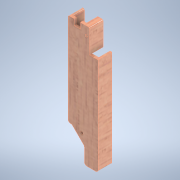
# Autodesk Inventor part: Case
Saved by Autodesk Inventor 2021 (Build 250183000, 183)
## iProperties
Created: 2021-02-15
Part Number: Case
Material: Holz (Eiche)
Document SubType Name: Modeling
Designer: nostrabis
Density: 0.76 g/cm^3
Appearance: Weißeiche - natur - mittlerer Glanz
Mass: 6.60677 g
Surface Area: 82.7336 cm^2
Volume: 8.69312 cm^3
Author: nostrabis
Autodesk Inventor part; units mm, degrees
ref_plane "YZ Plane" through (0, 0, 0) normal (1, 0, 0) x (0, 1, 0)
ref_plane "XZ Plane" through (0, 0, 0) normal (0, 1, 0) x (-1, 0, 0)
sketch "Skizze1" plane through (0, 0, 0) normal (0, 0, 1) x (1, 0, 0)
  point P0 (0, 0)
ref_plane "Arbeitsebene1" through (0, 0, 0) normal (0, 0, 1) x (1, 0, 0)
sketch "Skizze2" plane through (0, 0, 0) normal (0, 0, 1) x (1, 0, 0)
  line L0 (-10, -0.5) -> (-12, -0.5) projected
  line L1 (-12, -0.5) -> (-12, -23.5) projected
  arc A0 (-12, -23.5) -> (-10, -25.5) centre (-10, -23.5) ccw projected
  line L2 (-10, -25.5) -> (-9.8284, -25.5) projected
  arc A1 (-8.4142, -26.0858) -> (-9.8284, -25.5) centre (-9.8284, -27.5) ccw projected
  line L3 (0.4142, -34.9142) -> (-8.4142, -26.0858) projected
  arc A2 (1, -36.3284) -> (0.4142, -34.9142) centre (-1, -36.3284) ccw projected
  line L4 (1, -36.3284) -> (1, -46.5) projected
  arc A3 (1, -46.5) -> (3, -48.5) centre (3, -46.5) ccw projected
  line L5 (3, -48.5) -> (10, -48.5) projected
  arc A4 (10, -48.5) -> (12, -46.5) centre (10, -46.5) ccw projected
  line L6 (12, -46.5) -> (12, 31.5) projected
  line L7 (11, 32.5) -> (10, 32.5) projected
  line L8 (10, 32.5) -> (10, -46.5) projected
  line L9 (10, -46.5) -> (3, -46.5) projected
  line L10 (3, -46.5) -> (3, -23.5) projected
  line L11 (3, -23.5) -> (-10, -23.5) projected
  line L12 (-10, -23.5) -> (-10, -0.5) projected
  arc A5 (1, 48.5) -> (0, 47.5) centre (1, 47.5) ccw projected
  line L13 (0, 47.5) -> (0, 32.5) projected
  line L14 (0, 32.5) -> (5, 32.5) projected
  line L15 (5, 32.5) -> (5, 47.5) projected
  arc A6 (5, 47.5) -> (4, 48.5) centre (4, 47.5) ccw projected
  line L16 (4, 48.5) -> (1, 48.5) projected
  line L17 (-12, 12.5) -> (-10, 12.5) projected
  line L18 (-10, 12.5) -> (-10, 47.5) projected
  arc A7 (-10, 47.5) -> (-12, 47.5) centre (-11, 47.5) ccw projected
  line L19 (-12, 47.5) -> (-12, 12.5) projected
  line L20 (-10, 12.5) -> (-10, -0.5) projected
  line L21 (-12, 12.5) -> (-10, 12.5) projected
  line L22 (-12, -0.5) -> (-12, 12.5) projected
  line L23 (-10, -0.5) -> (-12, -0.5) projected
  arc A8 (12, 31.5) -> (11, 32.5) centre (11, 31.5) ccw projected
  point P0 (0, 0)
extrude "Extrusion1" add sketch "Skizze2" along normal blind 9
sketch "Skizze3" plane through (0, 0, 9) normal (0, 0, 1) x (1, 0, 0)
  line L0 (-12, 47.5) -> (-12, -23.5) projected
  arc A0 (-12, -23.5) -> (-10, -25.5) centre (-10, -23.5) ccw projected
  line L1 (-10, -25.5) -> (-9.8284, -25.5) projected
  arc A1 (-8.4142, -26.0858) -> (-9.8284, -25.5) centre (-9.8284, -27.5) ccw projected
  line L2 (-8.4142, -26.0858) -> (0.4142, -34.9142) projected
  arc A2 (1, -36.3284) -> (0.4142, -34.9142) centre (-1, -36.3284) ccw projected
  line L3 (1, -36.3284) -> (1, -46.5) projected
  arc A3 (1, -46.5) -> (3, -48.5) centre (3, -46.5) ccw projected
  line L4 (3, -48.5) -> (10, -48.5) projected
  arc A4 (10, -48.5) -> (12, -46.5) centre (10, -46.5) ccw projected
  line L5 (12, -46.5) -> (12, 31.5) projected
  line L6 (11, 32.5) -> (10, 32.5) projected
  line L7 (10, 32.5) -> (10, -46.5) projected
  line L8 (10, -46.5) -> (3, -46.5) projected
  line L9 (3, -46.5) -> (3, -23.5) projected
  line L10 (3, -23.5) -> (-10, -23.5) projected
  line L11 (-10, -23.5) -> (-10, 47.5) projected
  arc A5 (-10, 47.5) -> (-12, 47.5) centre (-11, 47.5) ccw projected
  line L12 (0, 32.5) -> (5, 32.5) projected
  line L13 (5, 32.5) -> (5, 47.5) projected
  arc A6 (5, 47.5) -> (4, 48.5) centre (4, 47.5) ccw projected
  line L14 (4, 48.5) -> (1, 48.5) projected
  arc A7 (1, 48.5) -> (0, 47.5) centre (1, 47.5) ccw projected
  line L15 (0, 47.5) -> (0, 32.5) projected
  line L16 (10, 32.5) -> (5, 32.5) projected
  line L17 (-11, 48.5) -> (4, 48.5)
  arc A8 (12, 31.5) -> (11, 32.5) centre (11, 31.5) ccw projected
  point P0 (0, 0)
  constraints: 2 end point, 1 horizontal, 1 other
extrude "Extrusion2" add sketch "Skizze3" along normal blind 2
sketch "Skizze5" plane through (-10, -23.5, 0) normal (1, 0, 0) x (0, 0, -1)
  line L0 (0, 0) -> (0, 71) projected
  line L1 (0, 71) -> (-9, 71) projected
  line L2 (-9, 0) -> (-9, 71) projected
  line L3 (0, 0) -> (-9, 0) projected
  line L4 (-9, 0) -> (-9, 71) projected
  line L5 (-9, 0) -> (-4, 0)
  line L6 (-4, 0) -> (-4, 5)
  line L7 (-4, 5) -> (-9, 5)
  line L8 (-9, 5) -> (-9, 0)
  point P0 (0, 23.5)
  point P1 (-9, 5)
  dimension "d4" = 5
  dimension "d5" = 5
  constraints: 8 end point, 2 parallel, 1 horizontal, 1 perpendicular
  measures "d4" distance of L7.end L6.end
  measures "d5" distance of L6.end L5.end
extrude "Extrusion3" add sketch "Skizze5" along normal blind 2.5 contours L3 L2 L7 L6
sketch "Skizze6" plane through (-7.5, -23.5, 0) normal (1, 0, 0) x (0, 0, -1)
  line L0 (-4, 0) -> (-4, 5) projected
  line L1 (-4, 0) -> (-9, 0) projected
  line L2 (-4, 5) -> (-9, 5)
  line L3 (-9, 5) -> (-9, 0)
  line L4 (-9, 0) -> (-4, 0)
  line L5 (-4, 0) -> (-4, 5)
  point P0 (0, 23.5)
  constraints: 8 end point, 2 parallel, 1 horizontal, 1 perpendicular
extrude "Extrusion4" cut sketch "Skizze6" against normal blind 1
sketch "Skizze7" plane through (0, 0, 0) normal (0, 0, -1) x (-1, 0, 0)
  line L0 (0, 32.5) -> (-5, 32.5) projected
  line L1 (0, 32.5) -> (-3.8, 32.5)
  line L2 (-3.8, 32.5) -> (-3.8, 34.5)
  line L3 (-3.8, 34.5) -> (0, 34.5)
  line L4 (0, 34.5) -> (0, 32.5)
  point P0 (0, 0)
  dimension "d10" = 2
  dimension "d11" = 3.8
  constraints: 8 end point, 2 parallel, 1 horizontal, 1 perpendicular
  measures "d10" distance of L1.end L2.end
  measures "d11" distance of L2.end L3.end
extrude "Extrusion5" cut sketch "Skizze7" against normal up to surface (9 mm away)
sketch "Skizze8" plane through (0, 0, 11) normal (0, 0, 1) x (1, 0, 0)
  line L0 (3.8, 32.5) -> (5, 32.5) projected
  line L1 (12, -46.5) -> (12, 31.5) projected
  line L2 (5, 32.5) -> (12, 32.5)
  line L3 (12, 32.5) -> (12, 29.5)
  line L4 (12, 29.5) -> (5, 29.5)
  line L5 (5, 29.5) -> (5, 32.5)
  point P0 (0, 0)
  dimension "d14" = 3
  constraints: 8 end point, 2 parallel, 1 horizontal, 1 perpendicular, 1 point on line
  measures "d14" distance of L2.end L3.end
extrude "Extrusion6" cut sketch "Skizze8" against normal through all
sketch "Skizze9" plane through (5, 32.5, 0) normal (0, -1, 0) x (1, 0, 0)
  line L0 (-1.2, 0) -> (-1.2, 9) projected
  line L1 (0, 0) -> (0, 11) projected
  line L2 (-1.2, 0) -> (0, 0)
  line L3 (0, 0) -> (0, 9)
  line L4 (0, 9) -> (-1.2, 9)
  line L5 (-1.2, 9) -> (-1.2, 0)
  point P0 (-5, 0)
  dimension "d17" = 9
  constraints: 8 end point, 2 parallel, 1 horizontal, 1 perpendicular, 1 point on line
  measures "d17" distance of L3.end L2.end
extrude "Extrusion7" add sketch "Skizze9" along normal blind 3
sketch "Skizze10" plane through (-12, -23.5, 0) normal (-1, 0, 0) x (0, 0, 1)
  line L0 (0, 0) -> (0, 71) projected
  line L1 (0, 23.8) -> (1.5, 23.8)
  line L2 (1.5, 23.8) -> (1.5, 38.5)
  line L3 (1.5, 38.5) -> (0, 38.5)
  line L4 (0, 38.5) -> (0, 23.8)
  line L5 (0, 71) -> (11, 71) projected
  point P0 (0, 23.5)
  point P1 (0, 38.5)
  dimension "d20" = 1.5
  dimension "d21" = 14.7
  dimension "d57" = 23.8
  constraints: 8 end point, 2 parallel, 1 horizontal, 1 perpendicular, 1 point on line
  measures "d20" distance of L2.end L3.end
  measures "d21" distance of L1.end L2.end
  measures "d57" distance from line of L1 L0.start
extrude "Extrusion8" cut sketch "Skizze10" against normal up to surface (22 mm away)
sketch "Skizze11" plane through (0, 0, 9) normal (0, 0, -1) x (-1, 0, 0)
  line L0 (-4, 48.5) -> (11, 48.5) projected
  line L1 (7.2, 48.5) -> (2.2, 48.5)
  line L2 (2.2, 48.5) -> (2.2, 43.6)
  line L3 (2.2, 43.6) -> (7.2, 43.6)
  line L4 (7.2, 43.6) -> (7.2, 48.5)
  line L5 (12, 47.5) -> (12, 15) projected
  point P0 (0, 0)
  point P1 (2.2, 48.5)
  dimension "d25" = 4.9
  dimension "d26" = 5
  dimension "d27" = 4.8
  constraints: 8 end point, 2 parallel, 1 horizontal, 1 perpendicular, 1 point on line
  measures "d25" distance between parallel lines of L3 L0
  measures "d26" distance of L2.end L3.end
  measures "d27" distance between parallel lines of L4 L5
extrude "Extrusion9" cut sketch "Skizze11" against normal blind 3
sketch "Skizze12" plane through (0, 0, 0) normal (0, 0, -1) x (-1, 0, 0)
  line L0 (-3, -23.5) -> (10, -23.5) projected
  line L1 (-3, -46.5) -> (-3, -23.5) projected
  point P0 (0, 0)
  point P1 (1, -27.5)
  dimension "d30" = 4
  dimension "d31" = 4
  measures "d30" distance from line of L0 point (1, -27.5)
  measures "d31" distance from line of L1 point (1, -27.5)
hole "Bohrung1" at (-1, -27.5, 0) direction (0, 0, 1) diameter 2 end through all
sketch "Skizze13" plane through (0, 0, 0) normal (0, 0, -1) x (-1, 0, 0)
  line L0 (-5, 29.5) -> (-5, 47.5) projected
  line L1 (-4, 48.5) -> (-1, 48.5) projected
  point P0 (0, 0)
  point P1 (-2.5, 41.5)
  dimension "d39" = 2.5
  dimension "d40" = 7
  measures "d39" distance from line of L0 point (-2.5, 41.5)
  measures "d40" distance from line of L1 point (-2.5, 41.5)
hole "Bohrung2" at (2.5, 41.5, 0) direction (0, 0, 1) diameter 2 end through all
sketch "Skizze14" plane through (-8.5, -23.5, 0) normal (1, 0, 0) x (0, 0, -1)
  line L0 (-9, 5) -> (-4, 5) projected
  line L1 (-4, 5) -> (-4, 0) projected
  point P0 (0, 23.5)
  point P1 (-6.5, 2.5)
  dimension "d48" = 2.5
  dimension "d49" = 2.5
  measures "d48" distance from line of L0 point (-6.5, 2.5)
  measures "d49" distance from line of L1 point (-6.5, 2.5)
hole "Bohrung3" at (-8.5, -21, 6.5) direction (-1, 0, 0) diameter 2.5 end through all
sketch "Skizze16" plane through (0, 0, 0) normal (0, 0, -1) x (-1, 0, 0)
  line L0 (-5, 29.5) -> (-10, 29.5) projected
  line L1 (-10, 29.5) -> (-10.5, 29.5)
  line L2 (-10.5, 29.5) -> (-10.5, 19.5)
  line L3 (-10.5, 19.5) -> (-10, 19.5)
  line L4 (-10, 19.5) -> (-10, 29.5)
  point P0 (0, 0)
  dimension "d63" = 0.5
  dimension "d64" = 10
  constraints: 8 end point, 2 parallel, 1 horizontal, 1 perpendicular
  measures "d63" distance of L3.end L2.end
  measures "d64" distance of L2.end L1.end
extrude "Extrusion11" cut sketch "Skizze16" against normal up to surface (9 mm away)
